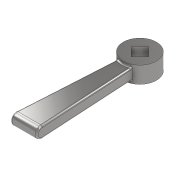
# Autodesk Inventor part: 手柄
Saved by Autodesk Inventor 2022 (Build 260153000, 153)
## iProperties
Created: 2023-03-14
Part Number: 手柄
Material: 不锈钢
Document SubType Name: Modeling
Designer: Lzy18
Density: 8 g/cm^3
Appearance: 半抛光
Author: Lzy18
Autodesk Inventor part; units mm, degrees
ref_plane "YZ Plane" through (0, 0, 0) normal (1, 0, 0) x (0, 1, 0)
ref_plane "XZ Plane" through (0, 0, 0) normal (0, 1, 0) x (-1, 0, 0)
ref_plane "XY Plane" through (0, 0, 0) normal (0, 0, 1) x (1, 0, 0)
sketch "草图1" plane through (0, 0, 0) normal (0, 1, 0) x (-1, 0, 0)
  circle A0 centre (0, 0) radius 20
  line L0 (16.1427, 140) -> (-15.8573, 140)
  line L1 (-15.8573, 140) -> (-8.8573, 17.9318)
  line L2 (9.1427, 17.7879) -> (16.1427, 140)
  line L3 (0.1427, 158.3232) -> (0.1427, -47.9442)
  circle A1 centre (-13.7393, 138) radius 2
  circle A2 centre (14.0249, 138) radius 2
  line L4 (-15.4558, 133) -> (15.7418, 133)
  point P0 (14.0249, 140)
  point P1 (-13.7393, 140)
  point P2 (-15.736, 137.8855)
  point P3 (16.0216, 137.8856)
  dimension "d0" = 40
  dimension "d1" = 32
  dimension "d3" = 140
  dimension "d4" = 16
  dimension "d5" = 18
  dimension "d6" = 9
  dimension "d7" = 4
  dimension "d8" = 4
  dimension "d16" = 7
  constraints: 10 end point, 4 tangent, 3 centre point, 2 horizontal, 2 point on circle, 2 point on line, 2 vertical, 1 coincident
  measures "d0" diameter of A0
  measures "d1" distance of L0.start L0.end
  measures "d3" distance from line of L0 point (0, 0)
  measures "d4" distance from line of L0.start L3
  measures "d5" horizontal distance of L1.end L2.start
  measures "d6" distance from line of L3 L2.start
  measures "d7" diameter of A1
  measures "d8" diameter of A2
  measures "d16" distance between parallel lines of L4 L0
sketch "草图2" plane through (0, 0, 0) normal (0, 1, 0) x (-1, 0, 0)
  circle A0 centre (0, 0) radius 20
  line L0 (0, -10.6066) -> (-10.6066, 0)
  line L1 (-10.6066, 0) -> (0, 10.6066)
  line L2 (0, 10.6066) -> (10.6066, 0)
  line L3 (10.6066, 0) -> (0, -10.6066)
  dimension "d11" = 40
  dimension "d12" = 7.5
  constraints: 8 end point, 2 coincident, 1 centre point, 9 other
  measures "d11" diameter of A0
  measures "d12" distance from line of L3 point (0, 0)
extrude "拉伸2" add sketch "草图2" along normal mid plane 20
extrude "拉伸4" add sketch "草图1" along normal mid plane 14 contours A0 L3 L4 L2 | A0 L1 L4 L3
sketch "草图6" plane through (0, 0, 0) normal (1, 0, 0) x (0, 1, 0)
  circle A0 centre (0, 133) radius 7
  point P0 (0, 0)
  dimension "d27" = 14
  constraints: 1 centre point
  measures "d27" diameter of A0
extrude "拉伸7" add sketch "草图6" along normal up to surface surface through (15.4558, 0, 133) normal (0.9983598, 0, -0.0572509)
sketch "草图7" plane through (0, 0, 0) normal (-1, 0, 0) x (0, 0, 1)
  line L0 (133, -7) -> (133, 7) projected
  arc A0 (133, -7) -> (133, 7) centre (133, 0) ccw projected
  point P0 (0, 0)
extrude "拉伸8" add sketch "草图7" along normal up to surface surface through (-9.1427, 0, 17.7879) normal (-0.9983637, 0, -0.0571838)
fillet "圆角3" radius 2 8 edges at (-16.1427, 0, 140) (-12.4423, 7, 75.394) (-12.4423, -7, 75.394) (15.8573, 0, 140) (12.1566, 7, 75.4659) (12.1566, -7, 75.4659) (-0.1598, -7, 19.9994) (-0.1598, 7, 19.9994)
